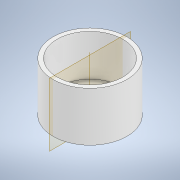
# Autodesk Inventor part: wheel
Saved by Autodesk Inventor 2022 (Build 260153000, 153)
## iProperties
Created: 2021-09-22
Part Number: wheel
Material: ABS プラスチック
Document SubType Name: Modeling
Designer: shiok
Density: 1.06 g/cm^3
Appearance: 滑らか - 白
Mass: 0.891598 g
Surface Area: 17.006 cm^2
Volume: 0.841131 cm^3
Author: shiok
Autodesk Inventor part; units mm, degrees
ref_plane "XZ Plane" through (0, 0, 0) normal (0, 1, 0) x (-1, 0, 0)
ref_plane "XY Plane" through (0, 0, 0) normal (0, 0, 1) x (1, 0, 0)
sketch "スケッチ6" plane through (0, 0, 0) normal (0, 1, 0) x (-1, 0, 0)
  arc A0 (9, 0) -> (-4.5, 7.7942) centre (0, 0) ccw
  line L0 (0, 0) -> (-4.5, 7.7942) construction
  line L1 (0, 0) -> (9, 0) construction
  arc A1 (8, 0) -> (-4, 6.9282) centre (0, 0) ccw
  line L2 (0, 0) -> (-4, 6.9282) construction
  line L3 (0, 0) -> (8, 0) construction
  arc A2 (7, 0) -> (-3.5, 6.0622) centre (0, 0) ccw
  line L4 (0, 0) -> (-3.5, 6.0622) construction
  line L5 (0, 0) -> (7, 0) construction
  arc A3 (4.7, 0) -> (-2.35, 4.0703) centre (0, 0) ccw
  arc A4 (3.5, 0) -> (-1.75, 3.0311) centre (0, 0) ccw
  line L6 (4.5041, 1.3429) -> (6.7082, 2)
  arc A5 (10.9533, 0) -> (5.4767, 9.4859) centre (0, 0) ccw
  line L7 (0, 0) -> (5.4767, 9.4859) construction
  line L8 (0, 0) -> (10.9533, 0) construction
  line L9 (-1.0891, 4.5721) -> (-1.6221, 6.8095)
  line L10 (0, 0) -> (9, 0)
  line L11 (0, 0) -> (-4.5, 7.7942)
  point P0 (-1.6221, 6.8095)
  point P1 (-4, 6.9282)
  point P2 (-1.75, 3.0311)
  dimension "d33" = 9
  dimension "d34" = 120
  dimension "d35" = 120
  dimension "d36" = 1
  dimension "d37" = 120
  dimension "d38" = 2
  dimension "d39" = 4.7
  dimension "d40" = 3.5
  dimension "d41" = 2
  dimension "d42" = 60
  constraints: 24 end point, 14 point on circle, 6 centre point, 6 coincident, 5 point on line, 3 collinear, 2 midpoint, 2 symmetric about line, 1 horizontal
  measures "d33" radius of A0
  measures "d34" angle of L1 L0
  measures "d35" angle of L3 L2
  measures "d36" radial gap between concentric circles of A0 A1
  measures "d37" angle of L5 L4
  measures "d38" radial gap between concentric circles of A0 A2
  measures "d39" radius of A3
  measures "d40" radius of A4
  measures "d41" distance from line of L5 L6.end
  measures "d42" angle of L8 L7
extrude "押し出し6" add sketch "スケッチ6" along normal blind 1.9 contours L10 A2 L11 A1 | L10 A3 L6 A2 | A2 L9 A3 L11 | L6 A3 L9 A2 | L10 A4 L11 A3
sketch "スケッチ7" plane through (0, 0, 0) normal (0, -1, 0) x (1, 0, 0)
  arc A0 (4, 6.9282) -> (-8, 0) centre (0, 0) ccw projected
  arc A1 (4.5, 7.7942) -> (-9, 0) centre (0, 0) ccw
  arc A2 (4, 6.9282) -> (-8, 0) centre (0, 0) ccw
  line L0 (0, 0) -> (4, 6.9282) construction
  line L1 (0, 0) -> (-8, 0) construction
  line L2 (4.5, 7.7942) -> (4, 6.9282)
  line L3 (-9, 0) -> (-8, 0)
  dimension "d45" = 120
  dimension "d46" = 9
  dimension "d47" = 8
  dimension "d48" = 120
  constraints: 8 end point, 4 point on circle, 2 centre point, 2 coincident, 1 horizontal
  measures "d46" radius of A1
  measures "d47" radius of A2
  measures "d48" angle of L0 L1
extrude "押し出し7" add sketch "スケッチ7" against normal blind 12
pattern_circular "円形状パターン1" count 3 over 360 about axis through (0, 0, 0) along (0, 1, 0)
sketch "スケッチ9" plane through (0, 0, 0) normal (0, -1, 0) x (1, 0, 0)
  circle A0 centre (0, 0) radius 4.5
  circle A1 centre (0, 0) radius 3.5 projected
  dimension "d62" = 9
  constraints: 1 centre point, 1 coincident
  measures "d62" diameter of A0
extrude "押し出し9" add sketch "スケッチ9" along normal blind 2
sketch "スケッチ11" plane through (0, 0, 0) normal (1, 0, 0) x (0, 1, 0)
  line L0 (0, 4.5) -> (-2, 4.5) projected
  circle A0 centre (-0.25, 4.5) radius 0.25
  line L1 (0, 9) -> (0, -9) projected
  point P0 (0, 0)
  point P1 (-0.5, 4.5)
  dimension "d73" = 0.5
  constraints: 1 centre point, 1 point on line, 1 tangent
  measures "d73" diameter of A0
sketch3d "3D スケッチ1"
  arc A0 (4.5, 0, 0) -> (0, 0, -4.5) centre (0, 0, 0) ccw
  arc A1 (0, 0, -4.5) -> (-4.5, 0, 0) centre (0, 0, 0) ccw
  arc A2 (-4.5, 0, 0) -> (0, 0, 4.5) centre (0, 0, 0) ccw
  arc A3 (0, 0, 4.5) -> (4.5, 0, 0) centre (0, 0, 0) ccw
sweep "スイープ1" cut profiles "スケッチ11" path "3D スケッチ1" picked at (-0.194, 4.3148) contours A0 L0
